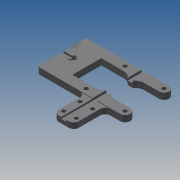
# Autodesk Inventor part: Drückbrücke_U
Saved by Autodesk Inventor 2015 SP1 (Build 190203100, 203)
## iProperties
Created: 2015-01-28
Part Number: Drückbrücke_U
Material: ABS-Kunststoff
Document SubType Name: Modeling
Designer: Marc
Density: 1.06 g/cm^3
Appearance: Gehont - dunkelgrau
Mass: 3.36639 g
Surface Area: 19.9083 cm^2
Volume: 3.17584 cm^3
Author: Marc
Autodesk Inventor part; units mm, degrees
ref_plane "YZ Plane" through (0, 0, 0) normal (1, 0, 0) x (0, 1, 0)
ref_plane "XZ Plane" through (0, 0, 0) normal (0, 1, 0) x (-1, 0, 0)
sketch "Skizze1" plane through (0, 0, 0) normal (0, 0, 1) x (1, 0, 0)
  line L0 (0, -27.3) -> (0, 27.3) projected
  line L1 (-71.7, 0) -> (34.7, 0) projected
  circle A0 centre (-15.5, 15.5) radius 1.55
  circle A1 centre (15.5, 15.5) radius 1.55
  circle A2 centre (-15.5, -15.5) radius 1.55
  circle A3 centre (15.5, -15.5) radius 1.55
  circle A4 centre (-16.5, 0) radius 11
  circle A5 centre (0, 0) radius 5.5
  circle A6 centre (-16.5, 0) radius 4
  arc A7 (-16.5, -7.5) -> (-16.5, 7.5) centre (-16.5, 0) ccw
  line L2 (-16.5, 7.5) -> (-36.5, 7.5)
  line L3 (-36.5, 7.5) -> (-56.5, 7.5)
  line L4 (-56.5, 7.5) -> (-56.5, -7.5)
  line L5 (-56.5, -7.5) -> (-16.5, -7.5)
  circle A8 centre (15.5, 15.5) radius 4
  circle A9 centre (-15.5, 15.5) radius 4
  line L6 (15.5, 11.5) -> (-15.5, 11.5)
  line L7 (15.5, 19.5) -> (-15.5, 19.5)
  line L8 (-15.5, 19.5) -> (-50.5, 19.5)
  line L9 (-15.5, 11.5) -> (-30.5, 11.5)
  line L10 (-50.5, 19.5) -> (-50.5, 0)
  line L11 (-30.5, 11.5) -> (-30.5, 0)
  line L12 (-15.5, -19.5) -> (-50.5, -19.5)
  line L13 (-15.5, -11.5) -> (-30.5, -11.5)
  line L14 (-50.5, -19.5) -> (-50.5, 0)
  line L15 (-30.5, -11.5) -> (-30.5, 0)
  line L16 (15.5, -11.5) -> (-15.5, -11.5)
  line L17 (15.5, -19.5) -> (-15.5, -19.5)
  line L18 (-15.5, -11.5) -> (15.5, -11.5)
  line L19 (15.5, -19.5) -> (-15.5, -19.5)
  line L20 (-30.5, -11.5) -> (15.5, -11.5)
  line L21 (15.5, -19.5) -> (-50.5, -19.5)
  arc A10 (15.5, -19.5) -> (15.5, -11.5) centre (15.5, -15.5) ccw
  point P0 (-50.5, 7.5)
  point P1 (-30.5, 7.5)
  dimension "d0" = 3.1
  dimension "d1" = 15.5
  dimension "d2" = 15.5
  dimension "d3" = 22
  dimension "d4" = 16.5
  dimension "d5" = 11
  dimension "d6" = 8
  dimension "d7" = 15
  dimension "d10" = 15
  dimension "d11" = 40
  dimension "d17" = 8
  dimension "d19" = 8
  dimension "d22" = 35
  dimension "d23" = 15
  constraints: 40 end point, 11 centre point, 9 symmetric about line, 8 point on circle, 6 coincident, 6 point on line, 5 horizontal, 4 tangent, 3 perpendicular, 1 collinear, 3 other
  measures "d0" diameter of A0
  measures "d1" distance from line of L1 A0.centre
  measures "d2" distance from line of L0 A0.centre
  measures "d3" diameter of A4
  measures "d4" distance from line of L0 A4.centre
  measures "d5" diameter of A5
  measures "d6" diameter of A6
  measures "d7" diameter of A7
  measures "d10" distance of L3.end L4.end
  measures "d11" distance from line of L2.start L4
  measures "d17" diameter of A8
  measures "d19" diameter of A9
  measures "d22" distance of L7.end L8.end
  measures "d23" distance of L6.end L9.end
ref_plane "Arbeitsebene1" through (0, 0, 5) normal (0, 0, 1) x (1, 0, 0)
extrude "Extrusion5" add sketch "Skizze1" along normal blind 5 contours L17 L12 L14 L5 L15 L13 L16 L0 | L0 L16 A10 L17 | L14 L1 L15 L5 | L10 L3 L2 L11 L1 | L6 A9 L7 L0 | L0 L7 A8 L6 | L2 L3 L10 L8 A9 L9 L11 | A8 | A9
sketch "Skizze4" plane through (0, 0, 5) normal (0, 0, 1) x (1, 0, 0)
  line L0 (-30.5, 11.5) -> (15.5, 11.5) projected
  arc A0 (15.5, 11.5) -> (15.5, 19.5) centre (15.5, 15.5) ccw projected
  line L1 (15.5, 19.5) -> (-50.5, 19.5) projected
  line L2 (-50.5, 19.5) -> (-50.5, -19.5) projected
  line L3 (-50.5, -19.5) -> (15.5, -19.5) projected
  arc A1 (15.5, -19.5) -> (15.5, -11.5) centre (15.5, -15.5) ccw projected
  line L4 (15.5, -11.5) -> (-30.5, -11.5) projected
  line L5 (-30.5, -11.5) -> (-30.5, 11.5) projected
  circle A2 centre (15.5, 15.5) radius 1.55 projected
  circle A3 centre (15.5, -15.5) radius 1.55 projected
  circle A4 centre (-15.5, -15.5) radius 1.55 projected
  circle A5 centre (-15.5, 15.5) radius 1.55 projected
  line L6 (-64.5, 0) -> (33.5, 0) projected
  line L7 (-30.5, -11.5) -> (-30.5, 11.5) projected
  line L8 (-50.5, -1.5) -> (-30.5, -1.5)
  line L9 (-30.5, -1.5) -> (-30.5, 1.5)
  line L10 (-30.5, 1.5) -> (-50.5, 1.5)
  line L11 (-50.5, 1.5) -> (-50.5, -1.5)
  point P0 (0, 0)
  dimension "d34" = 3
  constraints: 8 end point, 2 parallel, 2 point on line, 1 horizontal, 1 perpendicular, 1 other
  measures "d34" distance of L9.end L8.end
extrude "Extrusion8" cut sketch "Skizze4" against normal blind 1.5 contours L5 L6 L2 L10 | L5 L8 L2 L6
sketch "Skizze5" plane through (0, 0, 5) normal (0, 0, 1) x (1, 0, 0)
  line L0 (-50.5, 1.5) -> (-30.5, 1.5) projected
  line L1 (-30.5, 1.5) -> (-30.5, 11.5) projected
  line L2 (-30.5, 11.5) -> (15.5, 11.5) projected
  arc A0 (15.5, 11.5) -> (15.5, 19.5) centre (15.5, 15.5) ccw projected
  line L3 (15.5, 19.5) -> (-50.5, 19.5) projected
  line L4 (-50.5, 19.5) -> (-50.5, 1.5) projected
  circle A1 centre (15.5, 15.5) radius 1.55 projected
  circle A2 centre (-15.5, 15.5) radius 1.55 projected
  circle A3 centre (-15.5, -15.5) radius 1.55 projected
  circle A4 centre (15.5, -15.5) radius 1.55 projected
  line L5 (-30.5, -1.5) -> (-50.5, -1.5) projected
  line L6 (-50.5, -1.5) -> (-50.5, -19.5) projected
  line L7 (-50.5, -19.5) -> (15.5, -19.5) projected
  arc A5 (15.5, -19.5) -> (15.5, -11.5) centre (15.5, -15.5) ccw projected
  line L8 (15.5, -11.5) -> (-30.5, -11.5) projected
  line L9 (-30.5, -11.5) -> (-30.5, -1.5) projected
  line L10 (-30.5, -1.5) -> (-50.5, -1.5) projected
  line L11 (-30.5, 1.5) -> (-30.5, -1.5) projected
  line L12 (-50.5, 1.5) -> (-30.5, 1.5) projected
  line L13 (-50.5, -1.5) -> (-50.5, 1.5) projected
  line L14 (-64.5, 0) -> (33.5, 0) projected
  line L15 (-43.5, -2.75) -> (-41.1, -2.75)
  line L16 (-41.1, -2.75) -> (-41.1, 2.75)
  line L17 (-41.1, 2.75) -> (-43.5, 2.75)
  line L18 (-43.5, 2.75) -> (-43.5, -2.75)
  point P0 (0, 0)
  dimension "d37" = 2.4
  dimension "d38" = 5.5
  dimension "d39" = 7
  constraints: 8 end point, 2 parallel, 1 horizontal, 1 perpendicular, 1 other
  measures "d37" distance of L17.end L16.end
  measures "d38" distance of L16.end L15.end
  measures "d39" distance between parallel lines of L13 L18
extrude "Extrusion9" cut sketch "Skizze5" against normal blind 3.2 contours L18 L17 L16 L0 | L0 L16 L14 L18 | L14 L16 L5 L18 | L5 L16 L15 L18
sketch "Skizze6" plane through (0, 0, 5) normal (0, 0, 1) x (1, 0, 0)
  line L0 (15.5, 19.5) -> (-50.5, 19.5) projected
  line L1 (-50.5, -19.5) -> (15.5, -19.5) projected
  line L2 (-6.4, 19.5) -> (-2.4, 19.5)
  line L3 (-2.4, 19.5) -> (-2.4, -19.5)
  line L4 (-2.4, -19.5) -> (-6.4, -19.5)
  line L5 (-6.4, -19.5) -> (-6.4, 19.5)
  line L6 (-41.1, -1.5) -> (-41.1, -2.75) projected
  line L7 (-41.1, -2.75) -> (-43.5, -2.75) projected
  line L8 (-43.5, -2.75) -> (-43.5, -1.5) projected
  line L9 (-43.5, -1.5) -> (-50.5, -1.5) projected
  line L10 (-50.5, -1.5) -> (-50.5, -19.5) projected
  line L11 (-50.5, -19.5) -> (15.5, -19.5) projected
  arc A0 (15.5, -19.5) -> (15.5, -11.5) centre (15.5, -15.5) ccw projected
  line L12 (15.5, -11.5) -> (-30.5, -11.5) projected
  line L13 (-30.5, -11.5) -> (-30.5, -1.5) projected
  line L14 (-30.5, -1.5) -> (-41.1, -1.5) projected
  circle A1 centre (15.5, -15.5) radius 1.55 projected
  circle A2 centre (-15.5, -15.5) radius 1.55 projected
  line L15 (0, -27.3) -> (0, 27.3) projected
  line L16 (-64.5, 0) -> (33.5, 0) projected
  circle A3 centre (0, 0) radius 3.5191
  dimension "d42" = 4
  dimension "d43" = 2.4
  constraints: 8 end point, 2 parallel, 2 point on line, 1 centre point, 1 horizontal, 1 perpendicular, 1 other
  measures "d42" distance of L3.end L4.end
  measures "d43" distance between parallel lines of L15 L3
extrude "Extrusion10" cut sketch "Skizze6" against normal blind 1.9 contours L3 A3 L16 L5 L0 | L3 L16 A3 | L16 A3 L3 L12 L5 | L3 A3 L16 | L12 L3 L1 L5
fillet "Rundung1" radius 2 1 edges at (-50.5, -19.5, 2.5)
fillet "Rundung2" radius 2 1 edges at (-50.5, 19.5, 2.5)
sketch "Skizze11" plane through (0, 0, 5) normal (0, 0, 1) x (1, 0, 0)
  line L0 (-2.4, 11.5) -> (-6.4, 11.5) projected
  line L1 (-2.4, 19.5) -> (-2.4, 11.5) projected
  line L2 (-6.4, 19.5) -> (-2.4, 19.5) projected
  line L3 (-6.4, 11.5) -> (-6.4, 19.5) projected
  arc A0 (-48.5, 19.5) -> (-50.5, 17.5) centre (-48.5, 17.5) ccw projected
  line L4 (-50.5, 17.5) -> (-50.5, 1.5) projected
  line L5 (-50.5, 1.5) -> (-43.5, 1.5) projected
  line L6 (-43.5, 1.5) -> (-43.5, 2.75) projected
  line L7 (-43.5, 2.75) -> (-41.1, 2.75) projected
  line L8 (-41.1, 2.75) -> (-41.1, 1.5) projected
  line L9 (-41.1, 1.5) -> (-30.5, 1.5) projected
  line L10 (-30.5, 1.5) -> (-30.5, 11.5) projected
  line L11 (-30.5, 11.5) -> (-6.4, 11.5) projected
  line L12 (-6.4, 11.5) -> (-6.4, 19.5) projected
  line L13 (-6.4, 19.5) -> (-48.5, 19.5) projected
  circle A1 centre (-15.5, 15.5) radius 1.55 projected
  line L14 (-2.4, 19.5) -> (-2.4, 11.5) projected
  line L15 (-2.4, 11.5) -> (15.5, 11.5) projected
  arc A2 (15.5, 11.5) -> (15.5, 19.5) centre (15.5, 15.5) ccw projected
  line L16 (15.5, 19.5) -> (-2.4, 19.5) projected
  circle A3 centre (15.5, 15.5) radius 1.55 projected
  circle A4 centre (-15.5, -15.5) radius 1.55 projected
  arc A5 (-50.5, -17.5) -> (-48.5, -19.5) centre (-48.5, -17.5) ccw projected
  line L17 (-48.5, -19.5) -> (-6.4, -19.5) projected
  line L18 (-6.4, -19.5) -> (-6.4, -11.5) projected
  line L19 (-6.4, -11.5) -> (-30.5, -11.5) projected
  line L20 (-30.5, -11.5) -> (-30.5, -1.5) projected
  line L21 (-30.5, -1.5) -> (-41.1, -1.5) projected
  line L22 (-41.1, -1.5) -> (-41.1, -2.75) projected
  line L23 (-41.1, -2.75) -> (-43.5, -2.75) projected
  line L24 (-43.5, -2.75) -> (-43.5, -1.5) projected
  line L25 (-43.5, -1.5) -> (-50.5, -1.5) projected
  line L26 (-50.5, -1.5) -> (-50.5, -17.5) projected
  line L27 (-6.4, -11.5) -> (-2.4, -11.5) projected
  line L28 (-6.4, -19.5) -> (-6.4, -11.5) projected
  line L29 (-2.4, -19.5) -> (-6.4, -19.5) projected
  line L30 (-2.4, -11.5) -> (-2.4, -19.5) projected
  line L31 (-2.4, -11.5) -> (-2.4, -19.5) projected
  line L32 (-2.4, -19.5) -> (15.5, -19.5) projected
  arc A6 (15.5, -19.5) -> (15.5, -11.5) centre (15.5, -15.5) ccw projected
  line L33 (15.5, -11.5) -> (-2.4, -11.5) projected
  circle A7 centre (15.5, -15.5) radius 1.55 projected
  line L34 (-6.4, 11.5) -> (-6.4, 8.5)
  line L35 (-6.4, 8.5) -> (-2.4, 8.5)
  line L36 (-2.4, 8.5) -> (-2.4, 11.5)
  line L37 (-30.5, 11.5) -> (-6.4, 11.5) projected
  arc A8 (-6.4, 8.5) -> (-12.4, 11.5) centre (-12.6481, 3.5038) ccw
  line L38 (-30.5, 11.5) -> (15.5, 11.5) projected
  arc A9 (3.6, 11.5) -> (-2.4, 8.5) centre (3.8481, 3.5038) ccw
  line L39 (-65.3971, 0) -> (35.9828, 0) projected
  line L40 (-6.4, -11.5) -> (-6.4, -8.5)
  line L41 (-6.4, -8.5) -> (-2.4, -8.5)
  line L42 (-2.4, -8.5) -> (-2.4, -11.5)
  arc A10 (-12.4, -11.5) -> (-6.4, -8.5) centre (-12.6481, -3.5038) ccw
  arc A11 (-2.4, -8.5) -> (3.6, -11.5) centre (3.8481, -3.5038) ccw
  circle A12 centre (0, 0) radius 12 projected
  line L43 (-12.4, 11.5) -> (3.6, 11.5)
  line L44 (-12.4, -11.5) -> (3.6, -11.5)
  line L45 (15.5, -11.5) -> (-30.5, -11.5) projected
  point P0 (0, 0)
  dimension "d61" = 3
  dimension "d62" = 4
  dimension "d63" = 8
  dimension "d64" = 8
  dimension "d65" = 6
  dimension "d66" = 6
  constraints: 16 end point, 9 point on circle, 8 symmetric about line, 4 centre point, 3 point on line, 2 collinear, 1 perpendicular, 1 vertical, 2 other
  measures "d61" distance of L0.end L34.end
  measures "d62" distance of L34.end L35.end
  measures "d63" radius of A8
  measures "d64" radius of A9
  measures "d65" distance from line of L34 A8.end
  measures "d66" distance from line of L36 L43.end
extrude "Extrusion13" add sketch "Skizze11" against normal blind 5 contours L36 L35 L34 A12 L0 | L15 A12 A9 L36 | A12 L34 L0 | L15 A9 A12 | L34 A12 A8 L11 | L34 A8 A12 | A12 L33 L42 A11 | A11 L33 A12 | A12 L40 L19 A10 | A10 L40 A12 | L42 L27 A12 L40 L41 | A12 L27 L40
sketch "Skizze12" plane through (0, 0, 5) normal (0, 0, 1) x (1, 0, 0)
  line L0 (-2.4, 11.5) -> (-6.4, 11.5) projected
  line L1 (-2.4, 19.5) -> (-2.4, 11.5) projected
  line L2 (-6.4, 19.5) -> (-2.4, 19.5) projected
  line L3 (-6.4, 11.5) -> (-6.4, 19.5) projected
  line L4 (-6.4, -11.5) -> (-2.4, -11.5) projected
  line L5 (-6.4, -19.5) -> (-6.4, -11.5) projected
  line L6 (-2.4, -19.5) -> (-6.4, -19.5) projected
  line L7 (-2.4, -11.5) -> (-2.4, -19.5) projected
  line L8 (-6.4, -11.5) -> (-2.4, -11.5)
  line L9 (-2.4, -11.5) -> (-2.4, 11.5)
  line L10 (-2.4, 11.5) -> (-6.4, 11.5)
  line L11 (-6.4, 11.5) -> (-6.4, -11.5)
  point P0 (0, 0)
  constraints: 8 end point, 2 parallel, 1 horizontal, 1 perpendicular
extrude "Extrusion14" cut sketch "Skizze12" against normal blind 1.9 contours L9 L4 L11 L0
sketch "Skizze13" plane through (0, 0, 5) normal (0, 0, 1) x (1, 0, 0)
  line L0 (-41.1, 1.5) -> (-41.1, -1.5) projected
  line L1 (-30.5, -1.5) -> (-41.1, -1.5) projected
  line L2 (-30.5, 1.5) -> (-30.5, -1.5) projected
  line L3 (-41.1, 1.5) -> (-30.5, 1.5) projected
  line L4 (-6.4, -19.5) -> (-6.4, -8.5) projected
  arc A0 (-12.4, -11.5) -> (-6.4, -8.5) centre (-12.6481, -3.5038) ccw projected
  line L5 (-12.4, -11.5) -> (-30.5, -11.5) projected
  line L6 (-30.5, -11.5) -> (-30.5, -1.5) projected
  line L7 (-30.5, -1.5) -> (-41.1, -1.5) projected
  line L8 (-41.1, -1.5) -> (-41.1, -2.75) projected
  line L9 (-41.1, -2.75) -> (-43.5, -2.75) projected
  line L10 (-43.5, -2.75) -> (-43.5, -1.5) projected
  line L11 (-43.5, -1.5) -> (-50.5, -1.5) projected
  line L12 (-50.5, -1.5) -> (-50.5, -17.5) projected
  arc A1 (-50.5, -17.5) -> (-48.5, -19.5) centre (-48.5, -17.5) ccw projected
  line L13 (-48.5, -19.5) -> (-6.4, -19.5) projected
  circle A2 centre (-15.5, -15.5) radius 1.55 projected
  circle A3 centre (-15.5, 15.5) radius 1.55 projected
  line L14 (-6.4, 8.5) -> (-6.4, 19.5) projected
  line L15 (-6.4, 19.5) -> (-48.5, 19.5) projected
  arc A4 (-48.5, 19.5) -> (-50.5, 17.5) centre (-48.5, 17.5) ccw projected
  line L16 (-50.5, 17.5) -> (-50.5, 1.5) projected
  line L17 (-50.5, 1.5) -> (-43.5, 1.5) projected
  line L18 (-43.5, 1.5) -> (-43.5, 2.75) projected
  line L19 (-43.5, 2.75) -> (-41.1, 2.75) projected
  line L20 (-41.1, 2.75) -> (-41.1, 1.5) projected
  line L21 (-41.1, 1.5) -> (-30.5, 1.5) projected
  line L22 (-30.5, 1.5) -> (-30.5, 11.5) projected
  line L23 (-30.5, 11.5) -> (-12.4, 11.5) projected
  arc A5 (-6.4, 8.5) -> (-12.4, 11.5) centre (-12.6481, 3.5038) ccw projected
  line L24 (-41.1, 1.5) -> (-30.5, 1.5) projected
  line L25 (-30.5, -1.5) -> (-39.5, -1.5)
  line L26 (-39.5, -1.5) -> (-39.5, 1.5)
  line L27 (-39.5, 1.5) -> (-30.5, 1.5)
  line L28 (-30.5, 1.5) -> (-30.5, -1.5)
  point P0 (0, 0)
  dimension "d71" = 9
  constraints: 8 end point, 2 parallel, 1 horizontal, 1 perpendicular, 1 point on line
  measures "d71" distance of L26.end L27.end
extrude "Extrusion15" add sketch "Skizze13" against normal blind 1.5 contours L3 L2 L1 L26
sketch "Skizze16" plane through (15.5, -19.5, 0) normal (0, -1, 0) x (1, 0, 0)
  line L0 (-11.9, 0) -> (-11.9, 5) projected
  line L1 (-64, 0) -> (-64, 5) projected
  line L2 (-64, 0) -> (0, 0) projected
  line L3 (0, 0) -> (0, 5) projected
  line L4 (-17.9, 5) -> (0, 5) projected
  line L5 (-17.9, 5) -> (-17.9, 3.1) projected
  line L6 (-17.9, 3.1) -> (-21.9, 3.1) projected
  line L7 (-21.9, 3.1) -> (-21.9, 5) projected
  line L8 (-64, 5) -> (-21.9, 5) projected
  line L9 (-17.9, 5) -> (-11.9, 5)
  line L10 (-11.9, 5) -> (-11.9, 0)
  line L11 (-11.9, 0) -> (-25.9, 0)
  line L12 (-64, 0) -> (0, 0) projected
  line L13 (-64, 5) -> (-21.9, 5) projected
  line L14 (-21.9, 5) -> (-27.9, 5)
  line L15 (-27.9, 5) -> (-27.9, 0)
  line L16 (-27.9, 0) -> (-25.9, 0)
  line L17 (-17.9, 5) -> (-17.9, 3.1)
  line L18 (-17.9, 3.1) -> (-21.9, 3.1)
  line L19 (-21.9, 3.1) -> (-21.9, 5)
  point P0 (-15.5, 0)
  dimension "d75" = 6
  constraints: 18 end point, 5 perpendicular, 3 point on line, 1 collinear, 1 vertical
  measures "d75" distance of L7.end L14.end
extrude "Extrusion16" add sketch "Skizze16" along normal blind 25 contours L2 L15 L8 L7 L6 L5 L4 L0
sketch "Skizze17" plane through (0, 0, 5) normal (0, 0, 1) x (1, 0, 0)
  line L0 (-2.4, -8.5) -> (-2.4, -44.5) projected
  line L1 (3.6, -44.5) -> (-2.4, -44.5) projected
  line L2 (3.6, -19.5) -> (3.6, -44.5) projected
  line L3 (3.6, -19.5) -> (15.5, -19.5) projected
  arc A0 (15.5, -19.5) -> (15.5, -11.5) centre (15.5, -15.5) ccw projected
  line L4 (15.5, -11.5) -> (3.6, -11.5) projected
  arc A1 (-2.4, -8.5) -> (3.6, -11.5) centre (3.8481, -3.5038) ccw projected
  circle A2 centre (15.5, -15.5) radius 1.55 projected
  circle A3 centre (-15.5, 15.5) radius 1.55 projected
  line L5 (-6.4, -44.5) -> (-6.4, -8.5) projected
  arc A4 (-12.4, -11.5) -> (-6.4, -8.5) centre (-12.6481, -3.5038) ccw projected
  line L6 (-12.4, -11.5) -> (-30.5, -11.5) projected
  line L7 (-30.5, -11.5) -> (-30.5, 11.5) projected
  line L8 (-30.5, 11.5) -> (-12.4, 11.5) projected
  arc A5 (-6.4, 8.5) -> (-12.4, 11.5) centre (-12.6481, 3.5038) ccw projected
  line L9 (-6.4, 8.5) -> (-6.4, 19.5) projected
  line L10 (-6.4, 19.5) -> (-48.5, 19.5) projected
  arc A6 (-48.5, 19.5) -> (-50.5, 17.5) centre (-48.5, 17.5) ccw projected
  line L11 (-50.5, 17.5) -> (-50.5, 1.5) projected
  line L12 (-50.5, 1.5) -> (-43.5, 1.5) projected
  line L13 (-43.5, 1.5) -> (-43.5, 2.75) projected
  line L14 (-43.5, 2.75) -> (-41.1, 2.75) projected
  line L15 (-41.1, 2.75) -> (-41.1, 1.5) projected
  line L16 (-41.1, 1.5) -> (-39.5, 1.5) projected
  line L17 (-39.5, 1.5) -> (-39.5, -1.5) projected
  line L18 (-39.5, -1.5) -> (-41.1, -1.5) projected
  line L19 (-41.1, -1.5) -> (-41.1, -2.75) projected
  line L20 (-41.1, -2.75) -> (-43.5, -2.75) projected
  line L21 (-43.5, -2.75) -> (-43.5, -1.5) projected
  line L22 (-43.5, -1.5) -> (-50.5, -1.5) projected
  line L23 (-50.5, -1.5) -> (-50.5, -17.5) projected
  arc A7 (-50.5, -17.5) -> (-48.5, -19.5) centre (-48.5, -17.5) ccw projected
  line L24 (-48.5, -19.5) -> (-12.4, -19.5) projected
  line L25 (-12.4, -19.5) -> (-12.4, -44.5) projected
  line L26 (-6.4, -44.5) -> (-12.4, -44.5) projected
  circle A8 centre (-15.5, -15.5) radius 1.55 projected
  circle A9 centre (0.6, -26.5) radius 1.5
  circle A10 centre (-9.4, -26.5) radius 1.5
  circle A11 centre (0.6, -39.5) radius 1.5
  circle A12 centre (-9.4, -39.5) radius 1.5
  point P0 (0, 0)
  dimension "d78" = 3
  dimension "d79" = 3
  dimension "d80" = 3
  dimension "d81" = 3
  dimension "d82" = 18
  dimension "d84" = 3
  dimension "d85" = 3
  dimension "d86" = 5
  constraints: 4 centre point, 2 horizontal alignment, 2 vertical alignment
  measures "d78" diameter of A9
  measures "d79" diameter of A10
  measures "d80" distance from line of L0 A9.centre
  measures "d81" distance from line of L5 A10.centre
  measures "d82" distance from line of L1 A9.centre
  measures "d84" diameter of A11
  measures "d85" diameter of A12
  measures "d86" distance from line of L1 A11.centre
extrude "Extrusion17" cut sketch "Skizze17" against normal blind 5 contours A9 | A10 | A11 | A12
sketch "Skizze18" plane through (15.5, -44.5, 0) normal (0, -1, 0) x (1, 0, 0)
  line L0 (-11.9, 0) -> (-11.9, 5) projected
  line L1 (-11.9, 5) -> (-17.9, 5) projected
  line L2 (-17.9, 5) -> (-17.9, 3.1) projected
  line L3 (-17.9, 3.1) -> (-21.9, 3.1) projected
  line L4 (-21.9, 3.1) -> (-21.9, 5) projected
  line L5 (-21.9, 5) -> (-27.9, 5) projected
  line L6 (-27.9, 5) -> (-27.9, 0) projected
  line L7 (-27.9, 0) -> (-11.9, 0) projected
  line L8 (-11.9, 5) -> (-11.9, 4.5)
  line L9 (-11.9, 5) -> (-11.9, 0) projected
  line L10 (-11.9, 4.5) -> (-27.9, 4.5)
  line L11 (-27.9, 5) -> (-27.9, 0) projected
  line L12 (-27.9, 4.5) -> (-27.9, 5)
  line L13 (-27.9, 5) -> (-11.9, 5)
  point P0 (-15.5, 0)
  dimension "d89" = 0.5
  constraints: 8 end point, 2 perpendicular, 2 point on line, 1 collinear
  measures "d89" distance of L0.end L8.end
extrude "Extrusion18" cut sketch "Skizze18" against normal blind 25 contours L10 L2 L1 L0 | L10 L4 L13 L2 | L6 L5 L4 L10
fillet "Rundung3" radius 4 1 edges at (3.6, -19.5, 2.25)
fillet "Rundung4" radius 4 3 edges at (-12.4, -19.5, 2.25) (-12.4, -44.5, 2.25) (3.6, -44.5, 2.25)
